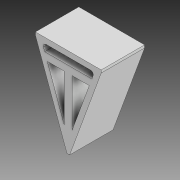
# Autodesk Inventor part: MainBracketT
Saved by Autodesk Inventor 2020 (Build 240168000, 168)
## iProperties
Created: 2021-01-14
Part Number: MainBracketT
Material: Generic
Document SubType Name: Modeling
Designer: DDeGo
Density: 1 g/cm^3
Appearance: Default
Author: DDeGo
Autodesk Inventor part; units mm, degrees
ref_plane "YZ Plane" through (0, 0, 0) normal (1, 0, 0) x (0, 1, 0)
ref_plane "XZ Plane" through (0, 0, 0) normal (0, 1, 0) x (-1, 0, 0)
ref_plane "XY Plane" through (0, 0, 0) normal (0, 0, 1) x (1, 0, 0)
sketch "Sketch1" plane through (0, 0, 0) normal (0, 0, 1) x (1, 0, 0)
  line L0 (0, 0) -> (0, 16.4748) construction
  line L1 (0, 16.4748) -> (-6.0643, 16.4748)
  line L2 (-6.0643, 16.4748) -> (-6.0643, 15.9748)
  line L3 (-6.0643, 15.9748) -> (-0.25, 0)
  line L4 (-0.25, 0) -> (0, 0)
  line L5 (0, 16.4748) -> (6.0643, 16.4748)
  line L6 (6.0643, 16.4748) -> (6.0643, 15.9748)
  line L7 (6.0643, 15.9748) -> (0.25, 0)
  line L8 (0.25, 0) -> (0, 0)
  line L9 (-4.1041, 15.4748) -> (-0.684, 15.4748)
  line L10 (-0.684, 15.4748) -> (4.1041, 15.4748)
  line L11 (4.574, 14.8038) -> (0.653, 4.031)
  line L12 (-0.653, 4.031) -> (-4.574, 14.8038)
  arc A0 (-4.1041, 15.4748) -> (-4.574, 14.8038) centre (-4.1041, 14.9748) ccw
  arc A1 (4.574, 14.8038) -> (4.1041, 15.4748) centre (4.1041, 14.9748) ccw
  arc A2 (-0.653, 4.031) -> (0.653, 4.031) centre (0, 4.2687) ccw
  line L13 (-4.4335, 14.1829) -> (3.654, 14.1829) construction
  line L14 (3.654, 14.1829) -> (3.654, 4.1829) construction
  line L15 (3.654, 4.1829) -> (-4.4335, 4.1829) construction
  line L16 (-4.4335, 4.1829) -> (-4.4335, 14.1829) construction
  line L17 (-0.752, 3.1829) -> (-0.752, 12.8814)
  line L18 (-0.752, 12.8814) -> (-4.4424, 12.8814)
  line L19 (-4.4424, 12.8814) -> (-4.4424, 14.1829)
  line L20 (-4.4424, 14.1829) -> (4.4004, 14.1829)
  line L21 (4.4004, 14.1829) -> (4.4004, 12.8814)
  line L22 (4.4004, 12.8814) -> (0.7099, 12.8814)
  line L23 (0.7099, 12.8814) -> (0.7099, 3.1829)
  line L24 (0.7099, 3.1829) -> (-0.752, 3.1829)
  point P0 (-4.8182, 15.4748)
  point P1 (4.8182, 15.4748)
  point P2 (0, 2.2369)
  dimension "d0" = 0.25
  dimension "d1" = 20
  dimension "d2" = 0.5
  dimension "d3" = 17
  dimension "d4" = 1
  dimension "d7" = 0.5
  constraints: 26 end point, 6 point on circle, 6 point on line, 6 tangent, 3 centre point, 3 symmetric about line, 2 perpendicular, 1 equal radius, 1 parallel, 1 vertical, 5 other
  measures "d0" distance of L3.end L0.start
  measures "d1" angle of L0 L3
  measures "d2" distance of L1.end L2.end
  measures "d3" distance of L2.end L3.end
  measures "d4" distance between parallel lines of L1 L9
  measures "d7" radius of A0
extrude "Extrusion1" add sketch "Sketch1" along normal blind 8 contours L5 L6 L7 L8 L4 L3 L2 L1 | L20 L11 L22 L23 A2 L12 L17 L18 | L12 L18 L19 L20 | L20 L21 L22 L11 | L12 A2 L11 L23 L24 L17
body "Solid1"
